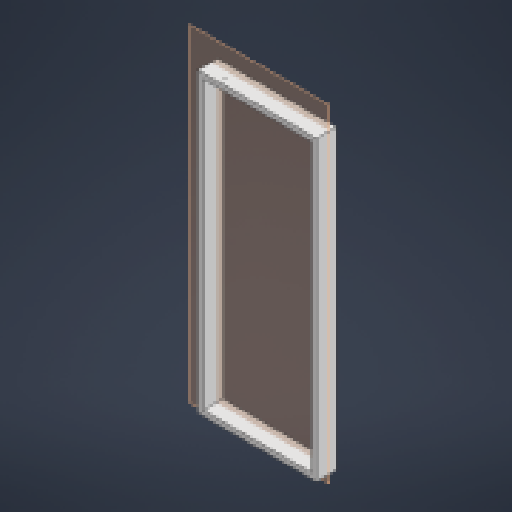
# Autodesk Inventor part: DoorFrame
Saved by Autodesk Inventor 2026.2 (Build 302298000, 298)
## iProperties
Created: 2026-03-06
Part Number: DoorFrame
Material: Generic
Document SubType Name: Modeling
Designer: brand
Density: 1 g/cm^3
Appearance: Default
Author: brand
Autodesk Inventor part; units mm, degrees
ref_plane "YZ Plane" through (0, 0, 0) normal (1, 0, 0) x (0, 1, 0)
ref_plane "XZ Plane" through (0, 0, 0) normal (0, 1, 0) x (-1, 0, 0)
ref_plane "XY Plane" through (0, 0, 0) normal (0, 0, 1) x (1, 0, 0)
ref_plane "Work Plane1" through (0, 0, 0) normal (0, 0, 1) x (1, 0, 0)
sketch "Sketch1" plane through (0, 0, 0) normal (0, 0, 1) x (1, 0, 0)
  line L0 (-295.275, -1057.275) -> (454.025, -1057.275) projected
  line L1 (454.025, -1057.275) -> (454.025, 962.025) projected
  circle A0 centre (384.175, -28.575) radius 31.4325 projected
  line L2 (454.025, 962.025) -> (-295.275, 962.025) projected
  line L3 (-295.275, 962.025) -> (-295.275, -1057.275) projected
  line L4 (462.153, 970.153) -> (462.153, -1065.403)
  line L5 (462.153, -1065.403) -> (-303.403, -1065.403)
  line L6 (-303.403, -1065.403) -> (-303.403, 970.153)
  line L7 (-303.403, 970.153) -> (462.153, 970.153)
  line L8 (500.253, -1103.503) -> (500.253, 1008.253)
  line L9 (500.253, 1008.253) -> (-341.503, 1008.253)
  line L10 (-341.503, 1008.253) -> (-341.503, -1103.503)
  line L11 (-341.503, -1103.503) -> (500.253, -1103.503)
  point P0 (-454.025, -1057.275)
  point P1 (454.025, 1057.275)
  point P2 (-454.025, 1057.275)
  point P3 (-454.025, 933.45)
  point P4 (-454.025, 819.15)
  point P5 (-454.025, 114.3)
  point P6 (-454.025, 0)
  point P7 (-454.025, -704.85)
  point P8 (-454.025, -819.15)
  dimension "d17" = 8.128
  dimension "d18" = 38.1
  constraints: 16 end point, 6 other
  measures "d17" distance between parallel lines of L1 L4
  measures "d18" distance between parallel lines of L4 L8
extrude "Extrusion1" add sketch "Sketch1" along normal blind 95.25 and the other way blind 44.45 contours L11 L10 L9 L8
sketch "Sketch2" plane through (-341.503, 1008.253, 95.25) normal (0, 1, 0) x (1, 0, 0)
  circle A0 centre (147.6845, 40.534) radius 3.175
  point P0 (341.503, 95.25)
  dimension "d19" = 6.35
  constraints: 3 coincident, 1 centre point, 1 other
  measures "d19" diameter of A0
extrude "Extrusion2" cut sketch "Sketch2" against normal blind 95.25
body "Solid1"
